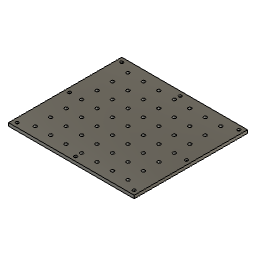
MFT Side (Autodesk Fusion 360 design; units mm, degrees)
Autodesk Fusion 360 part; units mm, degrees
sketch "Sketch1" plane through (0, 0, 0) normal (0, 0, 1) x (1, 0, 0)
  line L0 (390.525, -352) -> (-390.525, -352)
  line L1 (-390.525, -352) -> (-390.525, 352)
  line L2 (-390.525, 352) -> (390.525, 352)
  line L3 (390.525, 352) -> (390.525, -352)
  line L4 (390.525, -352) -> (-390.525, 352) construction
  line L5 (-390.525, -352) -> (390.525, 352) construction
  circle A0 centre (0, 0) radius 10
  circle A1 centre (-288, -288) radius 10
  circle A2 centre (-192, -288) radius 10
  circle A3 centre (-96, -288) radius 10
  circle A4 centre (0, -288) radius 10
  circle A5 centre (96, -288) radius 10
  circle A6 centre (192, -288) radius 10
  circle A7 centre (288, -288) radius 10
  circle A8 centre (-288, -192) radius 10
  circle A9 centre (-192, -192) radius 10
  circle A10 centre (-96, -192) radius 10
  circle A11 centre (0, -192) radius 10
  circle A12 centre (96, -192) radius 10
  circle A13 centre (192, -192) radius 10
  circle A14 centre (288, -192) radius 10
  circle A15 centre (-288, -96) radius 10
  circle A16 centre (-192, -96) radius 10
  circle A17 centre (-96, -96) radius 10
  circle A18 centre (0, -96) radius 10
  circle A19 centre (96, -96) radius 10
  circle A20 centre (192, -96) radius 10
  circle A21 centre (288, -96) radius 10
  circle A22 centre (-288, 0) radius 10
  circle A23 centre (-192, 0) radius 10
  circle A24 centre (-96, 0) radius 10
  circle A25 centre (96, 0) radius 10
  circle A26 centre (192, 0) radius 10
  circle A27 centre (288, 0) radius 10
  circle A28 centre (-288, 96) radius 10
  circle A29 centre (-192, 96) radius 10
  circle A30 centre (-96, 96) radius 10
  circle A31 centre (0, 96) radius 10
  circle A32 centre (96, 96) radius 10
  circle A33 centre (192, 96) radius 10
  circle A34 centre (288, 96) radius 10
  circle A35 centre (-288, 192) radius 10
  circle A36 centre (-192, 192) radius 10
  circle A37 centre (-96, 192) radius 10
  circle A38 centre (0, 192) radius 10
  circle A39 centre (96, 192) radius 10
  circle A40 centre (192, 192) radius 10
  circle A41 centre (288, 192) radius 10
  circle A42 centre (-288, 288) radius 10
  circle A43 centre (-192, 288) radius 10
  circle A44 centre (-96, 288) radius 10
  circle A45 centre (0, 288) radius 10
  circle A46 centre (96, 288) radius 10
  circle A47 centre (192, 288) radius 10
  circle A48 centre (288, 288) radius 10
  circle A49 centre (384, -288) radius 10
  circle A50 centre (384, -192) radius 10
  circle A51 centre (384, -96) radius 10
  circle A52 centre (384, 0) radius 10
  circle A53 centre (384, 96) radius 10
  circle A54 centre (384, 192) radius 10
  circle A55 centre (384, 288) radius 10
  dimension "d1" = 781.05
  dimension "d2" = 704
  dimension "d3" = 20
  dimension "d6" = 96
  dimension "d7" = 96
  constraint horizontal L0
  constraint perpendicular L0 L1
  constraint parallel L0 L2
  constraint parallel L1 L3
  constraint coincident L4 A0.centre
  constraint coincident L5 A0.centre
  constraint coincident A0.centre origin
  measures "d1" distance of L1.end L2.end
  measures "d2" distance of L0.end L1.end
  measures "d3" diameter of A0
extrude "Extrude1" add sketch "Sketch1" along normal blind 19.05 contours L0 L1 L2 L3 A49 A50 A51 A52 A53 A54 A55 | L3 A49 | L3 A50 | L3 A55 | L3 A51 | L3 A54 | L3 A52 | L3 A53 picked at (384.7263, -291.1646) picked at (379.6291, -189.2794) picked at (384.7263, 284.8354) picked at (385.0976, -95.2699) picked at (388.2662, 188.6677) picked at (386.0356, -2.4329) picked at (385.0976, 95.2699)
sketch "Sketch2" plane through (0, 0, 19.05) normal (0, 0, 1) x (-1, 0, 0)
  circle A0 centre (192, -288) radius 10
  circle A1 centre (-192, -288) radius 10
  circle A2 centre (96, 192) radius 10
  circle A3 centre (288, 192) radius 10
  circle A4 centre (0, 192) radius 10
  circle A5 centre (288, 96) radius 10
  circle A6 centre (96, 0) radius 10
  circle A7 centre (288, 0) radius 10
  circle A8 centre (192, 0) radius 10
  circle A9 centre (-192, 0) radius 10
  circle A10 centre (-288, 0) radius 10
  circle A11 centre (288, -96) radius 10
  circle A12 centre (-96, 0) radius 10
  circle A13 centre (-96, -288) radius 10
  circle A14 centre (192, 192) radius 10
  circle A15 centre (-288, -288) radius 10
  circle A16 centre (0, -288) radius 10
  circle A17 centre (-288, -192) radius 10
  circle A18 centre (192, -192) radius 10
  circle A19 centre (96, -192) radius 10
  circle A20 centre (288, -192) radius 10
  circle A21 centre (-288, -96) radius 10
  circle A22 centre (0, -96) radius 10
  circle A23 centre (-96, -96) radius 10
  circle A24 centre (-192, -96) radius 10
  circle A25 centre (-192, -192) radius 10
  circle A26 centre (-96, 96) radius 10
  circle A27 centre (-288, 96) radius 10
  circle A28 centre (-192, 96) radius 10
  circle A29 centre (0, 96) radius 10
  circle A30 centre (96, 96) radius 10
  circle A31 centre (192, 96) radius 10
  circle A32 centre (-96, 192) radius 10
  circle A33 centre (-192, 192) radius 10
  circle A34 centre (-288, 192) radius 10
  circle A35 centre (192, -96) radius 10
  circle A36 centre (288, -288) radius 10
  circle A37 centre (96, -96) radius 10
  circle A38 centre (96, -288) radius 10
  circle A39 centre (-96, -192) radius 10
  circle A40 centre (288, 288) radius 10
  circle A41 centre (-96, 288) radius 10
  circle A42 centre (192, 288) radius 10
  circle A43 centre (-192, 288) radius 10
  circle A44 centre (0, 0) radius 10
  circle A45 centre (0, 288) radius 10
  circle A46 centre (-288, 288) radius 10
  circle A47 centre (0, -192) radius 10
  circle A48 centre (96, 288) radius 10
  line L0 (-390.525, -352) -> (390.525, -352)
  line L1 (390.525, -352) -> (390.525, 352)
  line L2 (390.525, 352) -> (-390.525, 352)
  line L3 (-390.525, 352) -> (-390.525, -352)
  point P0 (363.525, -325)
  point P1 (0.025, -325)
  point P2 (-363.475, -325)
  point P3 (363.525, 0)
  point P4 (0.025, 0)
  point P5 (-363.475, 0)
  point P6 (363.525, 325)
  point P7 (0.025, 325)
  point P8 (-363.475, 325)
  dimension "d17" = 27
  dimension "d18" = 27
  dimension "d21" = 727
  dimension "d22" = 650
  measures "d17" distance of L0 P0
  measures "d18" distance of L1 P0
hole "Hole1" at (-363.525, 325, 19.05) at (-0.025, 325, 19.05) at (-363.525, 0, 19.05) at (-363.525, -325, 19.05) at (-0.025, -325, 19.05) at (363.475, -325, 19.05) at (363.475, 0, 19.05) at (363.475, 325, 19.05) direction (0, 0, -1) diameter 6.35 end through all counterbore diameter 19.05 counterbore depth 9.8425
equation "d8 = ( 3 / 4 ) * 1 in"
